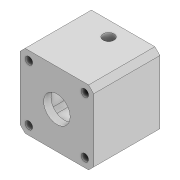
# Autodesk Inventor part: Part1
Saved by Autodesk Inventor 2021 (Build 250183000, 183)
## iProperties
Created: 2022-05-23
Part Number: Part1
Material: Generic
Document SubType Name: Modeling
Designer: romanp
Density: 1 g/cm^3
Appearance: Default
Author: romanp
Autodesk Inventor part; units mm, degrees
ref_plane "YZ Plane" through (0, 0, 0) normal (1, 0, 0) x (0, 1, 0)
ref_plane "XZ Plane" through (0, 0, 0) normal (0, 1, 0) x (-1, 0, 0)
ref_plane "XY Plane" through (0, 0, 0) normal (0, 0, 1) x (1, 0, 0)
sketch "Sketch11" plane through (0, 0, 0) normal (0, 0, 1) x (1, 0, 0)
  line L0 (-3.4593, 3.4593) -> (0, 0)
  line L1 (-3.4593, 3.4593) -> (-3.4593, 46.5407)
  line L2 (0, 50) -> (-3.4593, 46.5407)
  line L3 (43.0814, 50) -> (0, 50)
  line L4 (46.5407, 46.5407) -> (43.0814, 50)
  line L5 (46.5407, 3.4593) -> (46.5407, 46.5407)
  line L6 (43.0814, 0) -> (46.5407, 3.4593)
  line L7 (43.0814, 0) -> (0, 0)
  constraints: 16 end point
extrude "Extrusion8" add sketch "Sketch11" along normal blind 5
sketch "Sketch16" plane through (0, 0, 0) normal (0, 0, -1) x (-1, 0, 0)
  line L0 (-27.0407, 40) -> (-34.0407, 40)
  line L1 (-36.5407, 37.5) -> (-36.5407, 30.5)
  arc A0 (-34.0407, 40) -> (-36.5407, 37.5) centre (-34.0407, 37.5) ccw
  line L2 (-9.0407, 40) -> (-16.0407, 40)
  arc A1 (-6.5407, 37.5) -> (-9.0407, 40) centre (-9.0407, 37.5) ccw
  line L3 (-6.5407, 30.5) -> (-6.5407, 37.5)
  line L4 (-6.5407, 12.5) -> (-6.5407, 19.5)
  arc A2 (-9.0407, 10) -> (-6.5407, 12.5) centre (-9.0407, 12.5) ccw
  line L5 (-16.0407, 10) -> (-9.0407, 10)
  line L6 (-34.0407, 10) -> (-27.0407, 10)
  arc A3 (-36.5407, 12.5) -> (-34.0407, 10) centre (-34.0407, 12.5) ccw
  line L7 (-36.5407, 19.5) -> (-36.5407, 12.5)
  line L8 (0, 50) -> (3.4593, 46.5407) projected
  line L9 (-43.0814, 0) -> (-46.5407, 3.4593) projected
  line L10 (-46.5407, 46.5407) -> (-43.0814, 50) projected
  line L11 (-43.0814, 0) -> (-43.0814, 50)
  line L12 (3.4593, 3.4593) -> (0, 0) projected
  line L13 (-6.5407, 30.5) -> (-6.5407, 19.5)
  line L14 (-16.0407, 40) -> (-27.0407, 40)
  line L15 (-36.5407, 30.5) -> (-36.5407, 19.5)
  line L16 (-27.0407, 10) -> (-16.0407, 10)
  circle A4 centre (-2.5407, 44) radius 2.5
  circle A5 centre (-40.5407, 6) radius 2.5
  circle A6 centre (-2.5407, 6) radius 2.5
  circle A7 centre (-40.5407, 44) radius 2.5
  line L17 (0, 50) -> (3.4593, 46.5407)
  line L18 (3.4593, 46.5407) -> (3.4593, 3.4593) projected
  line L19 (0, 0) -> (-43.0814, 0) projected
  line L20 (3.4593, 3.4593) -> (0, 0)
  line L21 (0, 0) -> (-43.0814, 0)
  line L22 (-43.0814, 0) -> (-46.5407, 3.4593) projected
  line L23 (-43.0814, 0) -> (-46.5407, 3.4593)
  line L24 (-46.5407, 3.4593) -> (-46.5407, 46.5407) projected
  line L25 (-46.5407, 3.4593) -> (-46.5407, 46.5407)
  line L26 (-46.5407, 46.5407) -> (-43.0814, 50)
  line L27 (0, 50) -> (-43.0814, 50) projected
  line L28 (0, 50) -> (-43.0814, 50)
  dimension "d44" = 5
  dimension "d45" = 5
  dimension "d46" = 5
  dimension "d47" = 5
  constraints: 40 end point, 8 centre point, 8 collinear, 8 point on circle, 2 vertical, 1 perpendicular, 1 point on line
  measures "d44" diameter of A4
  measures "d45" diameter of A5
  measures "d46" diameter of A6
  measures "d47" diameter of A7
extrude "Extrusion11" add sketch "Sketch16" along normal blind 15
sketch "Sketch18" plane through (0, 0, -15) normal (0, 0, -1) x (-1, 0, 0)
  circle A0 centre (-2.5407, 6) radius 2.5 projected
  circle A1 centre (-2.5407, 6) radius 2.5
  circle A2 centre (-40.5407, 6) radius 2.5 projected
  circle A3 centre (-40.5407, 6) radius 2.5
  circle A4 centre (-40.5407, 44) radius 2.5 projected
  circle A5 centre (-40.5407, 44) radius 2.5
  circle A6 centre (-2.5407, 44) radius 2.5 projected
  circle A7 centre (-2.5407, 44) radius 2.5
  point P0 (0, 0)
  constraints: 4 centre point, 4 coincident
extrude "Extrusion12" cut sketch "Sketch18" against normal blind 100
sketch "Sketch19" plane through (0, 0, -15) normal (0, 0, -1) x (-1, 0, 0)
  circle A0 centre (-2.5407, 6) radius 2.5 projected
  circle A1 centre (-2.5407, 6) radius 4.3
  circle A2 centre (-40.5407, 6) radius 2.5 projected
  circle A3 centre (-40.5407, 6) radius 4.3
  circle A4 centre (-2.5407, 44) radius 2.5 projected
  circle A5 centre (-2.5407, 44) radius 4.3
  circle A6 centre (-40.5407, 44) radius 2.5 projected
  circle A7 centre (-40.5407, 44) radius 4.3
  point P0 (0, 0)
  dimension "d54" = 8.6
  dimension "d55" = 8.6
  dimension "d56" = 8.6
  dimension "d57" = 8.6
  constraints: 4 centre point, 4 coincident
  measures "d54" diameter of A1
  measures "d55" diameter of A3
  measures "d56" diameter of A5
  measures "d57" diameter of A7
extrude "Extrusion13" cut sketch "Sketch19" against normal blind 10 contours A0 | A1 | A2 | A3 | A5 | A6 | A7
sketch "Sketch20" plane through (0, 0, -15) normal (0, 0, -1) x (-1, 0, 0)
  line L0 (0, 50) -> (-43.0814, 50) projected
  line L1 (-43.0814, 50) -> (-46.5407, 46.5407) projected
  line L2 (-46.5407, 46.5407) -> (-46.5407, 3.4593) projected
  line L3 (-46.5407, 3.4593) -> (-43.0814, 0) projected
  line L4 (-43.0814, 0) -> (0, 0) projected
  line L5 (0, 0) -> (3.4593, 3.4593) projected
  line L6 (3.4593, 3.4593) -> (3.4593, 46.5407) projected
  line L7 (3.4593, 46.5407) -> (0, 50) projected
  circle A0 centre (-2.5407, 44) radius 4.3 projected
  circle A1 centre (-40.5407, 44) radius 4.3 projected
  circle A2 centre (-40.5407, 6) radius 4.3 projected
  circle A3 centre (-2.5407, 6) radius 4.3 projected
  arc A4 (-9.0407, 10) -> (-6.5407, 12.5) centre (-9.0407, 12.5) ccw projected
  line L8 (-9.0407, 10) -> (-34.0407, 10) projected
  line L9 (-36.5407, 12.5) -> (-36.5407, 37.5) projected
  arc A5 (-36.5407, 12.5) -> (-34.0407, 10) centre (-34.0407, 12.5) ccw projected
  line L10 (-6.5407, 37.5) -> (-6.5407, 12.5) projected
  arc A6 (-6.5407, 37.5) -> (-9.0407, 40) centre (-9.0407, 37.5) ccw projected
  line L11 (-34.0407, 40) -> (-9.0407, 40) projected
  arc A7 (-34.0407, 40) -> (-36.5407, 37.5) centre (-34.0407, 37.5) ccw projected
extrude "Extrusion14" add sketch "Sketch20" along normal blind 25
sketch "Sketch21" plane through (0, 50, 5) normal (0, 1, 0) x (1, 0, 0)
  line L0 (-1.7593, 45) -> (6.8407, 45) projected
  circle A0 centre (21.6907, 35) radius 2
  dimension "d63" = 4
  constraints: 1 centre point
  measures "d63" diameter of A0
extrude "Extrusion15" cut sketch "Sketch21" against normal blind 500
sketch "Sketch22" plane through (0, 50, 5) normal (0, 1, 0) x (1, 0, 0)
  circle A0 centre (21.6907, 35) radius 2 projected
  circle A1 centre (21.6907, 35) radius 3.75
  point P0 (0, 5)
  dimension "d67" = 7.5
  constraints: 1 centre point, 1 coincident
  measures "d67" diameter of A1
extrude "Extrusion16" cut sketch "Sketch22" against normal blind 5 contours A0 | A1
sketch "Sketch23" plane through (0, 0, 5) normal (0, -1, 0) x (1, 0, 0)
  circle A0 centre (21.6907, -35) radius 2 projected
  circle A1 centre (21.6907, -35) radius 3.75
  point P0 (0, -5)
  dimension "d70" = 7.5
  constraints: 1 centre point, 1 coincident
  measures "d70" diameter of A1
extrude "Extrusion17" cut sketch "Sketch23" against normal blind 5
sketch "Sketch25" plane through (0, 0, 5) normal (0, 0, 1) x (1, 0, 0)
  circle A0 centre (2.5407, 6) radius 2.5 projected
  circle A1 centre (40.5407, 44) radius 2.5 projected
  circle A2 centre (2.5407, 44) radius 2.5 projected
  circle A3 centre (40.5407, 6) radius 4.3 projected
  circle A4 centre (21.5407, 25) radius 9
  point P0 (0, 0)
  dimension "d75" = 18
  constraints: 1 centre point
  measures "d75" diameter of A4
extrude "Extrusion18" cut sketch "Sketch25" against normal blind 20 contours A4
sketch "Sketch26" plane through (0, 0, -40) normal (0, 0, -1) x (-1, 0, 0)
  circle A0 centre (-21.5407, 25) radius 9 projected
  arc A1 (-6.5407, 37.5) -> (-9.0407, 40) centre (-9.0407, 37.5) ccw projected
  line L0 (-9.0407, 40) -> (-34.0407, 40) projected
  arc A2 (-34.0407, 40) -> (-36.5407, 37.5) centre (-34.0407, 37.5) ccw projected
  line L1 (-36.5407, 37.5) -> (-36.5407, 12.5) projected
  arc A3 (-36.5407, 12.5) -> (-34.0407, 10) centre (-34.0407, 12.5) ccw projected
  line L2 (-34.0407, 10) -> (-9.0407, 10) projected
  arc A4 (-9.0407, 10) -> (-6.5407, 12.5) centre (-9.0407, 12.5) ccw projected
  line L3 (-6.5407, 12.5) -> (-6.5407, 37.5) projected
  circle A5 centre (-21.5407, 25) radius 9.144
  arc A6 (-6.3007, 37.7) -> (-8.8407, 40.24) centre (-8.8407, 37.7) ccw
  line L4 (-8.8407, 40.24) -> (-34.2407, 40.24)
  arc A7 (-34.2407, 40.24) -> (-36.7807, 37.7) centre (-34.2407, 37.7) ccw
  line L5 (-36.7807, 37.7) -> (-36.7807, 12.3)
  arc A8 (-36.7807, 12.3) -> (-34.2407, 9.76) centre (-34.2407, 12.3) ccw
  line L6 (-34.2407, 9.76) -> (-8.8407, 9.76)
  arc A9 (-8.8407, 9.76) -> (-6.3007, 12.3) centre (-8.8407, 12.3) ccw
  line L7 (-6.3007, 12.3) -> (-6.3007, 37.7)
  point P0 (0, 0)
  constraints: 8 end point, 8 point on circle, 5 centre point
extrude "Extrusion19" cut sketch "Sketch26" against normal blind 40 contours L7 A9 L6 A8 L5 A7 L4 A6
sketch "Sketch27" plane through (40.5407, 44, -5) normal (0, 0, -1) x (-1, 0, 0)
  circle A0 centre (38, -38) radius 2.5 projected
  circle A1 centre (38, -38) radius 4.3 projected
  circle A2 centre (0, -38) radius 2.5 projected
  circle A3 centre (0, -38) radius 4.3 projected
  circle A4 centre (0, 0) radius 2.5 projected
  circle A5 centre (0, 0) radius 4.3 projected
  circle A6 centre (38, 0) radius 4.3 projected
  circle A7 centre (38, 0) radius 2.5 projected
  point P0 (40.5407, -44)
extrude "Extrusion20" add sketch "Sketch27" along normal blind 2
sketch "Sketch28" plane through (0, 0, -40) normal (0, 0, -1) x (-1, 0, 0)
  arc A0 (-34.2407, 40.24) -> (-36.7807, 37.7) centre (-34.2407, 37.7) ccw projected
  line L0 (-34.2407, 40.24) -> (-8.8407, 40.24) projected
  arc A1 (-6.3007, 37.7) -> (-8.8407, 40.24) centre (-8.8407, 37.7) ccw projected
  line L1 (-6.3007, 37.7) -> (-6.3007, 12.3) projected
  arc A2 (-8.8407, 9.76) -> (-6.3007, 12.3) centre (-8.8407, 12.3) ccw projected
  line L2 (-8.8407, 9.76) -> (-34.2407, 9.76) projected
  arc A3 (-36.7807, 12.3) -> (-34.2407, 9.76) centre (-34.2407, 12.3) ccw projected
  line L3 (-36.7807, 12.3) -> (-36.7807, 37.7) projected
  line L4 (-43.0814, 50) -> (-46.5407, 46.5407) projected
  line L5 (-46.5407, 46.5407) -> (-46.5407, 3.4593) projected
  line L6 (-46.5407, 3.4593) -> (-43.0814, 0) projected
  line L7 (-43.0814, 0) -> (0, 0) projected
  line L8 (0, 0) -> (3.4593, 3.4593) projected
  line L9 (3.4593, 3.4593) -> (3.4593, 46.5407) projected
  line L10 (3.4593, 46.5407) -> (0, 50) projected
  line L11 (0, 50) -> (-43.0814, 50) projected
  circle A4 centre (-2.5407, 6) radius 4.3 projected
  circle A5 centre (-40.5407, 6) radius 4.3 projected
  circle A6 centre (-40.5407, 44) radius 4.3 projected
  circle A7 centre (-2.5407, 44) radius 4.3 projected
  arc A8 (-34.124, 40.1) -> (-36.6407, 37.5833) centre (-34.124, 37.5833) ccw
  line L12 (-34.124, 40.1) -> (-8.9574, 40.1)
  arc A9 (-6.4407, 37.5833) -> (-8.9574, 40.1) centre (-8.9574, 37.5833) ccw
  line L13 (-6.4407, 37.5833) -> (-6.4407, 12.4167)
  arc A10 (-8.9574, 9.9) -> (-6.4407, 12.4167) centre (-8.9574, 12.4167) ccw
  line L14 (-8.9574, 9.9) -> (-34.124, 9.9)
  arc A11 (-36.6407, 12.4167) -> (-34.124, 9.9) centre (-34.124, 12.4167) ccw
  line L15 (-36.6407, 12.4167) -> (-36.6407, 37.5833)
  circle A12 centre (-21.5407, 25) radius 9 projected
  circle A13 centre (-21.5407, 25) radius 8.9173
  constraints: 8 end point, 8 point on circle, 5 centre point, 1 coincident
extrude "Extrusion21" add sketch "Sketch28" against normal blind 40 contours L0 A1 L1 A2 L2 A3 L3 A0
sketch "Sketch29" plane through (21.6907, 5, -30) normal (0, -1, 0) x (1, 0, 0)
  circle A0 centre (0, 0) radius 2 projected
  circle A1 centre (0, 0) radius 2.05
  point P0 (-21.6907, 30)
  dimension "d86" = 4.1
  constraints: 1 centre point, 1 coincident
  measures "d86" diameter of A1
extrude "Extrusion22" cut sketch "Sketch29" against normal blind 100 contours A0 | A1
sketch "Sketch30" plane through (0, 0, -40) normal (0, 0, -1) x (-1, 0, 0)
  circle A0 centre (-2.5407, 44) radius 2.5 projected
  circle A1 centre (-2.5407, 44) radius 2.55
  circle A2 centre (-2.5407, 6) radius 4.3 projected
  circle A3 centre (-2.5407, 6) radius 2.55
  circle A4 centre (-40.5407, 6) radius 2.5 projected
  circle A5 centre (-40.5407, 6) radius 2.55
  circle A6 centre (-40.5407, 44) radius 2.5 projected
  circle A7 centre (-40.5407, 44) radius 2.55
  point P0 (0, 0)
  dimension "d89" = 5.1
  dimension "d90" = 5.1
  dimension "d91" = 5.1
  dimension "d92" = 5.1
  constraints: 4 centre point, 4 coincident
  measures "d89" diameter of A1
  measures "d90" diameter of A3
  measures "d91" diameter of A5
  measures "d92" diameter of A7
extrude "Extrusion23" cut sketch "Sketch30" against normal blind 100 contours A0 | A1 | A3 | A4 | A6 | A7
sketch "Sketch31" plane through (0, 0, -40) normal (0, 0, -1) x (-1, 0, 0)
  arc A0 (-34.2919, 40.3015) -> (-36.8422, 37.7513) centre (-34.2919, 37.7513) ccw
  line L0 (-34.2919, 40.3015) -> (-8.7894, 40.3015)
  arc A1 (-6.2392, 37.7512) -> (-8.7894, 40.3015) centre (-8.7895, 37.7512) ccw
  line L1 (-6.2392, 37.7512) -> (-6.2392, 12.2487)
  arc A2 (-8.7895, 9.6985) -> (-6.2392, 12.2487) centre (-8.7895, 12.2487) ccw
  line L2 (-8.7895, 9.6985) -> (-34.292, 9.6985)
  arc A3 (-36.8422, 12.2488) -> (-34.292, 9.6985) centre (-34.292, 12.2488) ccw
  line L3 (-36.8422, 12.2488) -> (-36.8422, 37.7513)
  circle A4 centre (-21.5407, 25) radius 9 projected
  circle A5 centre (-21.5407, 25) radius 1
  point P0 (0, 0)
  dimension "d95" = 2
  constraints: 8 end point, 8 point on circle, 5 centre point
  measures "d95" diameter of A5
extrude "Extrusion24" cut sketch "Sketch31" against normal blind 40 contours L0 A1 L1 A2 L2 A3 L3 A0 | A4 | A5
body "Solid2"
